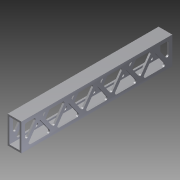
# Autodesk Inventor part: vertical frame piece2
Saved by Autodesk Inventor 2012 (Build 160160000, 160)
## iProperties
Created: 2013-01-04
Part Number: vertical frame piece2
Material: Default
Document SubType Name: Modeling
Designer: Bryce
Density: 1 g/cm^3
Author: Bryce
Autodesk Inventor part; units mm, degrees
ref_plane "YZ Plane" through (0, 0, 0) normal (1, 0, 0) x (0, 1, 0)
ref_plane "XZ Plane" through (0, 0, 0) normal (0, 1, 0) x (-1, 0, 0)
ref_plane "XY Plane" through (0, 0, 0) normal (0, 0, 1) x (1, 0, 0)
sketch "Sketch1" plane through (0, 0, 0) normal (0, 0, 1) x (1, 0, 0)
  line L0 (0, 0) -> (25.4, 0)
  line L1 (25.4, 0) -> (25.4, 50.8)
  line L2 (25.4, 50.8) -> (0, 50.8)
  line L3 (0, 50.8) -> (0, 0)
  line L4 (3.175, 3.175) -> (22.225, 3.175)
  line L5 (22.225, 3.175) -> (22.225, 47.625)
  line L6 (22.225, 47.625) -> (3.175, 47.625)
  line L7 (3.175, 47.625) -> (3.175, 3.175)
  dimension "d0" = 50.8
  dimension "d1" = 25.4
  dimension "d2" = 3.175
  dimension "d3" = 3.175
  dimension "d4" = 3.175
  dimension "d5" = 3.175
  constraints: 16 end point, 4 parallel, 2 horizontal, 2 perpendicular
  measures "d0" distance of L0.end L1.end
  measures "d1" distance of L1.end L2.end
  measures "d2" distance between parallel lines of L2 L6
  measures "d3" distance between parallel lines of L1 L5
  measures "d4" distance between parallel lines of L0 L4
  measures "d5" distance between parallel lines of L3 L7
extrude "Extrusion1" add sketch "Sketch1" along normal blind 279.4
sketch "Sketch2" plane through (25.4, 0, 0) normal (1, 0, 0) x (0, 0, -1)
  line L0 (-279.4, 50.8) -> (-279.4, 0) projected
  line L1 (0, 0) -> (-279.4, 0) projected
  line L2 (0, 50.8) -> (-279.4, 50.8) projected
  line L3 (-139.7, 0) -> (-139.7, 50.8)
  line L4 (-279.4, 50.8) -> (-139.7, 50.8)
  line L5 (-279.4, 50.8) -> (-279.4, 0)
  line L6 (-279.4, 0) -> (-139.7, 0)
  line L7 (-279.4, 0) -> (-279.4, 50.8)
  line L8 (-166.37, 11.8865) -> (-143.5756, 44.45)
  line L9 (-193.04, 38.9135) -> (-170.2456, 6.35)
  line L10 (-193.04, 44.45) -> (-166.37, 6.35) construction
  line L11 (-139.7, 6.35) -> (-139.7, 44.45)
  line L12 (-166.37, 6.35) -> (-139.7, 44.45) construction
  line L13 (-193.04, 38.9135) -> (-215.8344, 6.35)
  line L14 (-196.9156, 44.45) -> (-219.71, 11.8865)
  line L15 (-219.71, 6.35) -> (-193.04, 44.45) construction
  line L16 (-139.7, 44.45) -> (-273.05, 44.45)
  line L17 (-273.05, 6.35) -> (-139.7, 6.35)
  line L18 (-139.7, 0) -> (-279.4, 0)
  line L19 (-139.7, 50.8) -> (-279.4, 50.8)
  line L20 (-162.4944, 6.35) -> (-139.7, 38.9135)
  line L21 (-189.1644, 44.45) -> (-166.37, 11.8865)
  line L22 (-139.7, 50.8) -> (-139.7, 0)
  line L23 (-269.1744, 6.35) -> (-246.38, 38.9135)
  line L24 (-242.5044, 44.45) -> (-219.71, 11.8865)
  line L25 (-246.38, 44.45) -> (-219.71, 6.35) construction
  line L26 (-273.05, 44.45) -> (-273.05, 6.35)
  line L27 (-273.05, 11.8865) -> (-250.2556, 44.45)
  line L28 (-273.05, 6.35) -> (-246.38, 44.45) construction
  line L29 (-223.5856, 6.35) -> (-246.38, 38.9135)
  line L30 (0, 50.8) -> (0, 0)
  line L31 (-82.4844, 44.45) -> (-59.69, 11.8865)
  line L32 (0, 0) -> (-139.7, 0)
  line L33 (-139.7, 0) -> (0, 0)
  line L34 (-139.7, 50.8) -> (0, 50.8)
  line L35 (0, 50.8) -> (-139.7, 50.8)
  line L36 (-6.35, 6.35) -> (-139.7, 6.35)
  line L37 (-139.7, 44.45) -> (-6.35, 44.45)
  line L38 (-59.69, 6.35) -> (-86.36, 44.45) construction
  line L39 (-86.36, 38.9135) -> (-63.5656, 6.35)
  line L40 (0, 50.8) -> (0, 0)
  line L41 (0, 0) -> (0, 50.8)
  line L42 (-86.36, 44.45) -> (-113.03, 6.35) construction
  line L43 (-90.2356, 44.45) -> (-113.03, 11.8865)
  line L44 (-113.03, 11.8865) -> (-135.8244, 44.45)
  line L45 (-113.03, 6.35) -> (-139.7, 44.45) construction
  line L46 (-116.9056, 6.35) -> (-139.7, 38.9135)
  line L47 (-86.36, 38.9135) -> (-109.1544, 6.35)
  line L48 (-10.2256, 6.35) -> (-33.02, 38.9135)
  line L49 (-6.35, 44.45) -> (-6.35, 6.35)
  line L50 (-6.35, 11.8865) -> (-29.1444, 44.45)
  line L51 (-6.35, 6.35) -> (-33.02, 44.45) construction
  line L52 (-36.8956, 44.45) -> (-59.69, 11.8865)
  line L53 (-55.8144, 6.35) -> (-33.02, 38.9135)
  line L54 (-33.02, 44.45) -> (-59.69, 6.35) construction
  dimension "d8" = 34.992
  dimension "d9" = 69.984
  dimension "d10" = 69.984
  dimension "d11" = 69.984
  dimension "d12" = 69.984
  dimension "d13" = 3.175
  dimension "d14" = 3.175
  dimension "d15" = 3.175
  dimension "d16" = 3.175
  dimension "d17" = 3.175
  dimension "d18" = 3.175
  dimension "d19" = 3.175
  dimension "d20" = 3.175
  dimension "d21" = 3.175
  dimension "d22" = 3.175
  dimension "d23" = 6.35
  dimension "d24" = 6.35
  dimension "d25" = 0
  dimension "d26" = 6.35
  dimension "d27" = 139.7
  constraints: 96 end point, 27 symmetric about line, 8 parallel, 7 collinear, 3 point on line, 1 vertical, 40 other
  measures "d8" angle of L28 L26
  measures "d9" angle of L25 L28
  measures "d10" angle of L15 L25
  measures "d11" angle of L10 L15
  measures "d12" angle of L12 L10
  measures "d13" distance between parallel lines of L28 L27
  measures "d14" distance between parallel lines of L28 L23
  measures "d15" distance between parallel lines of L25 L29
  measures "d16" distance between parallel lines of L24 L25
  measures "d17" distance between parallel lines of L15 L14
  measures "d18" distance between parallel lines of L15 L13
  measures "d19" distance between parallel lines of L10 L9
  measures "d20" distance between parallel lines of L10 L21
  measures "d21" distance between parallel lines of L12 L8
  measures "d22" distance between parallel lines of L20 L12
  measures "d23" distance between parallel lines of L7 L26
  measures "d25" distance between parallel lines of L22 L11
  measures "d27" distance between parallel lines of L3 L0
extrude "Extrusion2" cut sketch "Sketch2" against normal blind 25.4 contours L17 L20 L3 | L3 L46 L36 | L8 L21 L16 | L37 L43 L44 | L17 L13 L9 | L47 L39 L36 | L14 L24 L16 | L37 L52 L31 | L17 L23 L29 | L53 L48 L36 | L27 L26 L16 | L37 L49 L50
fillet "Fillet1" radius 3.175 63 edges at (23.8125, 11.8865, 273.05) (23.8125, 44.45, 273.05) (23.8125, 44.45, 250.2556) (23.8125, 38.9135, 246.38) (23.8125, 6.35, 269.1744) (23.8125, 6.35, 223.5856) (23.8125, 11.8865, 219.71) (23.8125, 44.45, 242.5044) (23.8125, 44.45, 196.9156) (23.8125, 38.9135, 193.04) (23.8125, 6.35, 215.8344) (23.8125, 6.35, 170.2456) (23.8125, 11.8865, 166.37) (23.8125, 44.45, 189.1644) (23.8125, 44.45, 143.5756) (23.8125, 38.9135, 139.7) (1.5875, 6.35, 116.9056) (23.8125, 6.35, 116.9056) (23.8125, 6.35, 162.4944) (23.8125, 44.45, 135.8244) (23.8125, 11.8865, 113.03) (23.8125, 44.45, 90.2356) (23.8125, 38.9135, 86.36) (23.8125, 6.35, 109.1544) (23.8125, 6.35, 63.5656) (23.8125, 11.8865, 59.69) (23.8125, 44.45, 82.4844) (23.8125, 44.45, 36.8956) (23.8125, 38.9135, 33.02) (23.8125, 6.35, 55.8144) (23.8125, 6.35, 10.2256) (23.8125, 44.45, 29.1444) (23.8125, 44.45, 6.35) (23.8125, 11.8865, 6.35) (1.5875, 11.8865, 273.05) (1.5875, 44.45, 250.2556) (1.5875, 44.45, 273.05) (1.5875, 38.9135, 246.38) (1.5875, 6.35, 223.5856) (1.5875, 6.35, 269.1744) (1.5875, 6.35, 215.8344) (1.5875, 38.9135, 193.04) (1.5875, 6.35, 170.2456) (1.5875, 11.8865, 166.37) (1.5875, 44.45, 189.1644) (1.5875, 44.45, 143.5756) (1.5875, 6.35, 162.4944) (1.5875, 38.9135, 139.7) (1.5875, 11.8865, 113.03) (1.5875, 44.45, 135.8244) (1.5875, 44.45, 90.2356) (1.5875, 38.9135, 86.36) (1.5875, 6.35, 109.1544) (1.5875, 6.35, 63.5656) (1.5875, 11.8865, 59.69) (1.5875, 44.45, 82.4844) (1.5875, 44.45, 36.8956) (1.5875, 6.35, 55.8144) (1.5875, 6.35, 10.2256) (1.5875, 38.9135, 33.02) (1.5875, 44.45, 29.1444) (1.5875, 44.45, 6.35) (1.5875, 11.8865, 6.35)
equation "\"d2\" = d3"
equation "\"d3\" = d4"
equation "\"d4\" = d5"
equation "\"d9\" = 2 * d8"
equation "\"d10\" = d9"
equation "\"d11\" = d10"
equation "\"d12\" = d11"
equation "\"d14\" = d13"
equation "\"d15\" = d14"
equation "\"d16\" = d15"
equation "\"d17\" = d16"
equation "\"d18\" = d17"
equation "\"d19\" = d18"
equation "\"d20\" = d18"
equation "\"d21\" = d20"
equation "\"d22\" = d21"
body "Solid1"
